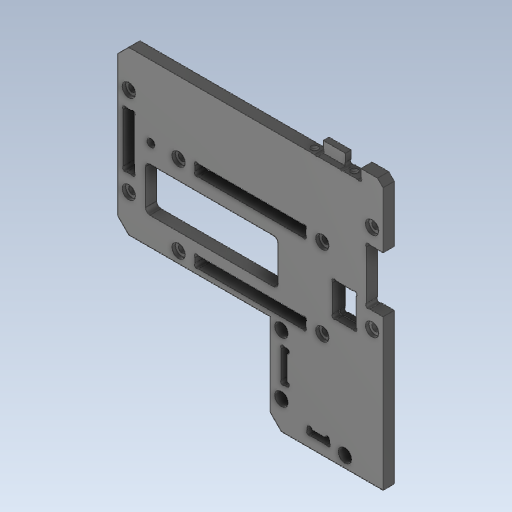
# Autodesk Inventor part: Cockpit_side_frame
Saved by Autodesk Inventor 2020.4 (Build 244396000, 396)
## iProperties
Part Number: Cockpit_side_frame
Material: アセタール樹脂、黒
Document SubType Name: Modeling
Designer: Masato Kubotera
Density: 1.425 g/cm^3
Appearance: 滑らか - 黒
Mass: 60.6497 g
Surface Area: 236.441 cm^2
Volume: 42.5612 cm^3
Description: POM T5
Author: Masato Kubotera
Autodesk Inventor part; units mm, degrees
ref_plane "YZ Plane" through (0, 0, 0) normal (1, 0, 0) x (0, 1, 0)
ref_plane "XZ Plane" through (0, 0, 0) normal (0, 1, 0) x (-1, 0, 0)
ref_plane "XY Plane" through (0, 0, 0) normal (0, 0, 1) x (1, 0, 0)
sketch "スケッチ1" plane through (0, 0, 0) normal (0, 1, 0) x (-1, 0, 0)
  line L0 (-60, 36.75) -> (60, 36.75) construction
  line L1 (60, 36.75) -> (60, -36.75) construction
  line L2 (60, -36.75) -> (-60, -36.75) construction
  line L3 (-60, -36.75) -> (-60, 36.75) construction
  line L4 (-60, 36.75) -> (60, -36.75) construction
  line L5 (60, 36.75) -> (-60, -36.75) construction
  line L6 (-52.5, 6.75) -> (52.5, 6.75) construction
  line L7 (52.5, 6.75) -> (52.5, 1.75) construction
  line L8 (52.5, 1.75) -> (-52.5, 1.75) construction
  line L9 (-52.5, 1.75) -> (-52.5, 6.75) construction
  line L10 (-52.5, 6.75) -> (52.5, 1.75) construction
  line L11 (52.5, 6.75) -> (-52.5, 1.75) construction
  line L12 (0, 36.75) -> (0, -36.75) construction
  line L13 (-57.5, 34.25) -> (-52.5, 34.25) construction
  line L14 (-52.5, 34.25) -> (-52.5, -34.25) construction
  line L15 (-52.5, -34.25) -> (-57.5, -34.25) construction
  line L16 (-57.5, -34.25) -> (-57.5, 34.25) construction
  line L17 (-57.5, 34.25) -> (-52.5, -34.25) construction
  line L18 (-52.5, 34.25) -> (-57.5, -34.25) construction
  line L19 (-55, 36.75) -> (-60, 31.75)
  line L20 (-60, 0) -> (60, 0) construction
  line L21 (-46.5, 41.75) -> (32.5, 41.75) construction
  line L22 (32.5, 41.75) -> (32.5, 11.75) construction
  line L23 (32.5, 11.75) -> (-46.5, 11.75) construction
  line L24 (-46.5, 11.75) -> (-46.5, 41.75) construction
  line L25 (-46.5, 41.75) -> (32.5, 11.75) construction
  line L26 (32.5, 41.75) -> (-46.5, 11.75) construction
  line L27 (-55, -36.75) -> (-60, -31.75)
  line L28 (-60, 31.75) -> (-60, -31.75)
  line L29 (55, -36.75) -> (60, -31.75) construction
  line L30 (-52.5, -29.25) -> (52.5, -29.25) construction
  line L31 (52.5, -29.25) -> (52.5, -34.25) construction
  line L32 (52.5, -34.25) -> (-52.5, -34.25) construction
  line L33 (-52.5, -34.25) -> (-52.5, -29.25) construction
  line L34 (-52.5, -29.25) -> (52.5, -34.25) construction
  line L35 (52.5, -29.25) -> (-52.5, -34.25) construction
  line L36 (-25, -29.25) -> (-25, -34.25) construction
  line L37 (-55, -34.25) -> (-55, 34.25) construction
  line L38 (-57.5, 12.5) -> (-52.5, 12.5) construction
  line L39 (-57.55, 12.55) -> (-52.45, 12.55)
  line L40 (-52.45, 12.55) -> (-52.45, -12.55)
  line L41 (-52.45, -12.55) -> (-57.55, -12.55)
  line L42 (-57.55, -12.55) -> (-57.55, 12.55)
  line L43 (-57.55, 12.55) -> (-52.45, -12.55) construction
  line L44 (-52.45, 12.55) -> (-57.55, -12.55) construction
  arc A0 (-52.45, 11.0651) -> (-53.9349, 12.55) centre (-53.1925, 11.8075) ccw
  circle A1 centre (-55, 20) radius 1.6
  circle A2 centre (-55, -20) radius 1.6
  arc A3 (-53.9349, -12.55) -> (-52.45, -11.0651) centre (-53.1925, -11.8075) ccw
  line L45 (-57.5, -12.5) -> (-52.5, -12.5) construction
  arc A4 (-56.0651, 12.55) -> (-57.55, 11.0651) centre (-56.8075, 11.8075) ccw
  arc A5 (-57.55, -11.0651) -> (-56.0651, -12.55) centre (-56.8075, -11.8075) ccw
  line L46 (-52.5, -31.75) -> (52.5, -31.75) construction
  line L47 (-25.05, -34.3) -> (-25.05, -29.2)
  line L48 (-25.05, -29.2) -> (25.05, -29.2)
  circle A6 centre (-32.5, -31.75) radius 1.6
  circle A7 centre (32.5, -31.75) radius 1.6
  line L49 (25, -29.25) -> (25, -34.25) construction
  line L50 (52.5, 36.75) -> (57.5, 36.75) construction
  line L51 (57.5, 36.75) -> (57.5, -34.25) construction
  line L52 (57.5, -34.25) -> (52.5, -34.25) construction
  line L53 (52.5, -34.25) -> (52.5, 36.75) construction
  line L54 (52.5, 36.75) -> (57.5, -34.25) construction
  line L55 (57.5, 36.75) -> (52.5, -34.25) construction
  line L56 (52.5, 1.25) -> (57.5, 1.25) construction
  line L57 (52.5, -11.25) -> (57.5, -11.25) construction
  line L58 (55, -34.25) -> (55, 36.75) construction
  circle A8 centre (55, -18.75) radius 1.6
  line L59 (60, -11.3) -> (52.45, -11.3)
  line L60 (52.45, -11.3) -> (52.45, 13.8)
  arc A9 (52.45, -9.8151) -> (53.9349, -11.3) centre (53.1925, -10.5575) ccw
  line L61 (52.5, 13.75) -> (57.5, 13.75) construction
  circle A10 centre (55, 21.25) radius 1.6
  line L62 (60, 13.8) -> (52.45, 13.8)
  arc A11 (53.9349, 13.8) -> (52.45, 12.3151) centre (53.1925, 13.0575) ccw
  arc A12 (-23.5651, -29.2) -> (-25.05, -30.6849) centre (-24.3075, -29.9425) ccw
  arc A13 (25.05, -30.6849) -> (23.5651, -29.2) centre (24.3075, -29.9425) ccw
  circle A14 centre (-55, 20) radius 3
  circle A15 centre (-32.5, -31.75) radius 3
  circle A16 centre (-55, -20) radius 3
  circle A17 centre (32.5, -31.75) radius 3
  line L63 (25.05, -34.3) -> (25.05, -29.2)
  line L64 (25.05, 6.8) -> (-25.05, 6.8)
  line L65 (-25.05, 6.8) -> (-25.05, 1.7)
  line L66 (-25.05, 1.7) -> (25.05, 1.7)
  line L67 (25.05, 1.7) -> (25.05, 6.8)
  line L68 (25.05, 6.8) -> (-25.05, 1.7) construction
  line L69 (-25.05, 6.8) -> (25.05, 1.7) construction
  line L70 (-25, 6.75) -> (-25, 1.75) construction
  arc A18 (-23.5651, 6.8) -> (-25.05, 5.3151) centre (-24.3075, 6.0575) ccw
  line L71 (52.5, 4.25) -> (-52.5, 4.25) construction
  circle A19 centre (-32.5, 4.25) radius 1.6
  line L72 (25, 6.75) -> (25, 1.75) construction
  arc A20 (25.05, 5.3151) -> (23.5651, 6.8) centre (24.3075, 6.0575) ccw
  circle A21 centre (32.5, 4.25) radius 1.6
  arc A22 (-25.05, 3.1849) -> (-23.5651, 1.7) centre (-24.3075, 2.4425) ccw
  arc A23 (23.5651, 1.7) -> (25.05, 3.1849) centre (24.3075, 2.4425) ccw
  line L73 (60, 31.75) -> (60, 13.8)
  line L74 (60, -11.3) -> (60, -31.75)
  circle A24 centre (-32.5, 4.25) radius 3
  circle A25 centre (55, -18.75) radius 3
  circle A26 centre (55, 21.25) radius 3
  circle A27 centre (32.5, 4.25) radius 3
  line L75 (60, 31.75) -> (60, 39.25)
  line L76 (21, 36.75) -> (-55, 36.75)
  line L77 (60, 39.25) -> (57.5, 41.75)
  line L78 (57.5, 41.75) -> (50, 41.75)
  line L79 (50, 41.75) -> (50, 36.75)
  line L80 (50, 36.75) -> (40.5, 36.75)
  line L81 (40.5, 36.75) -> (40.5, 41.75)
  line L82 (40.5, 41.75) -> (30.5, 41.75)
  line L83 (30.5, 41.75) -> (30.5, 36.75)
  line L84 (30.5, 36.75) -> (21, 36.75)
  line L85 (21, 36.75) -> (21, 36.75)
  circle A28 centre (-45, 4.25) radius 1.75
  line L86 (35.5, 41.75) -> (35.5, 36.75) construction
  line L87 (37.9, -8.6) -> (47.1, -8.6) construction
  line L88 (47.1, -8.6) -> (47.1, -22.4) construction
  line L89 (47.1, -22.4) -> (37.9, -22.4) construction
  line L90 (37.9, -22.4) -> (37.9, -8.6) construction
  line L91 (37.9, -8.6) -> (47.1, -22.4) construction
  line L92 (47.1, -8.6) -> (37.9, -22.4) construction
  line L93 (37.2, -7.95) -> (47.8, -7.95) construction
  line L94 (47.8, -7.95) -> (47.8, -23.05) construction
  line L95 (47.8, -23.05) -> (37.2, -23.05) construction
  line L96 (37.2, -23.05) -> (37.2, -7.95) construction
  line L97 (37.2, -7.95) -> (47.8, -23.05) construction
  line L98 (47.8, -7.95) -> (37.2, -23.05) construction
  line L99 (42.5, -7.95) -> (42.5, -23.05) construction
  line L100 (47.8, -15.5) -> (37.2, -15.5) construction
  line L101 (38.6349, -7.9) -> (46.3651, -7.9)
  line L102 (37.15, -9.3849) -> (37.15, -21.6151)
  line L103 (39.3349, -8.55) -> (45.6651, -8.55)
  line L104 (37.85, -10.0349) -> (37.85, -20.9651)
  arc A29 (38.6349, -7.9) -> (37.15, -9.3849) centre (37.8925, -8.6425) ccw
  arc A30 (39.3349, -8.55) -> (37.85, -10.0349) centre (38.5925, -9.2925) ccw
  arc A31 (47.85, -9.3849) -> (46.3651, -7.9) centre (47.1075, -8.6425) ccw
  arc A32 (47.15, -10.0349) -> (45.6651, -8.55) centre (46.4075, -9.2925) ccw
  line L105 (38.6349, -23.1) -> (46.3651, -23.1)
  line L106 (39.3349, -22.45) -> (45.6651, -22.45)
  arc A33 (37.15, -21.6151) -> (38.6349, -23.1) centre (37.8925, -22.3575) ccw
  arc A34 (37.85, -20.9651) -> (39.3349, -22.45) centre (38.5925, -21.7075) ccw
  arc A35 (46.3651, -23.1) -> (47.85, -21.6151) centre (47.1075, -22.3575) ccw
  arc A36 (45.6651, -22.45) -> (47.15, -20.9651) centre (46.4075, -21.7075) ccw
  line L107 (47.85, -9.3849) -> (47.85, -21.6151)
  line L108 (47.15, -10.0349) -> (47.15, -20.9651)
  line L109 (-45.5, -4.25) -> (10.5, -4.25)
  line L110 (12.5, -6.25) -> (12.5, -22.25)
  line L111 (10.5, -24.25) -> (-45.5, -24.25)
  line L112 (-47.5, -22.25) -> (-47.5, -6.25)
  line L113 (-47.5, -4.25) -> (12.5, -24.25) construction
  line L114 (12.5, -4.25) -> (-47.5, -24.25) construction
  arc A37 (-45.5, -4.25) -> (-47.5, -6.25) centre (-45.5, -6.25) ccw
  arc A38 (-47.5, -22.25) -> (-45.5, -24.25) centre (-45.5, -22.25) ccw
  arc A39 (10.5, -24.25) -> (12.5, -22.25) centre (10.5, -22.25) ccw
  arc A40 (12.5, -6.25) -> (10.5, -4.25) centre (10.5, -6.25) ccw
  line L115 (26.5, 36.75) -> (26.5, 32.75) construction
  line L116 (24.5, 32.75) -> (28.5, 32.75) construction
  line L117 (28.5, 32.75) -> (28.5, 36.75) construction
  line L118 (24.5, 32.75) -> (24.5, 36.75) construction
  line L119 (44.5, 36.75) -> (44.5, 32.75) construction
  line L120 (46.5, 32.75) -> (42.5, 32.75) construction
  line L121 (42.5, 32.75) -> (42.5, 36.75) construction
  line L122 (46.5, 32.75) -> (46.5, 36.75) construction
  arc A41 (48.5151, 36.75) -> (50, 38.2349) centre (49.2575, 37.4925) ccw
  arc A42 (29.0151, 36.75) -> (30.5, 38.2349) centre (29.7575, 37.4925) ccw
  arc A43 (40.5, 38.2349) -> (41.9849, 36.75) centre (41.2425, 37.4925) ccw
  line L123 (30.5, 36.75) -> (40.5, 36.75)
  line L124 (60, -36.75) -> (60, -79.25)
  line L125 (60, -79.25) -> (14, -79.25)
  line L126 (9, -74.25) -> (9, -36.75)
  arc A44 (-25.05, -32.8151) -> (-23.5651, -34.3) centre (-24.3075, -33.5575) ccw
  arc A45 (23.5651, -34.3) -> (25.05, -32.8151) centre (24.3075, -33.5575) ccw
  line L127 (60, -36.75) -> (60, -31.75)
  line L128 (-25.05, -34.3) -> (25.05, -34.3)
  line L129 (-55, -36.75) -> (9, -36.75)
  line L130 (16.5, -48.75) -> (50.5, -48.75) construction
  line L131 (50.5, -48.75) -> (50.5, -71.75) construction
  line L132 (50.5, -71.75) -> (16.5, -71.75) construction
  line L133 (16.5, -71.75) -> (16.5, -48.75) construction
  line L134 (16.5, -48.75) -> (50.5, -71.75) construction
  line L135 (50.5, -48.75) -> (16.5, -71.75) construction
  line L136 (14, -45.5) -> (16.5, -45.5) construction
  line L137 (16.5, -45.5) -> (16.5, -60.5) construction
  line L138 (16.5, -60.5) -> (14, -60.5) construction
  line L139 (14, -60.5) -> (14, -45.5) construction
  line L140 (14, -45.5) -> (16.5, -60.5) construction
  line L141 (16.5, -45.5) -> (14, -60.5) construction
  line L142 (13.95, -45.45) -> (16.55, -45.45)
  line L143 (16.55, -45.45) -> (16.55, -60.55)
  line L144 (16.55, -60.55) -> (13.95, -60.55)
  line L145 (13.95, -60.55) -> (13.95, -45.45)
  line L146 (13.95, -45.45) -> (16.55, -60.55) construction
  line L147 (16.55, -45.45) -> (13.95, -60.55) construction
  line L148 (15.25, -45.5) -> (15.25, -60.5) construction
  line L149 (14, -53) -> (16.5, -53) construction
  arc A46 (15.4349, -45.45) -> (13.95, -46.9349) centre (14.6925, -46.1925) ccw
  arc A47 (16.55, -47.55) -> (16.55, -45.45) centre (16.55, -46.5) ccw
  arc A48 (13.95, -59.0651) -> (15.4349, -60.55) centre (14.6925, -59.8075) ccw
  arc A49 (16.55, -60.55) -> (16.55, -58.45) centre (16.55, -59.5) ccw
  line L150 (11.5, -34.25) -> (16.5, -34.25) construction
  line L151 (16.5, -34.25) -> (16.5, -71.75) construction
  line L152 (16.5, -71.75) -> (11.5, -71.75) construction
  line L153 (11.5, -71.75) -> (11.5, -34.25) construction
  line L154 (11.5, -34.25) -> (16.5, -71.75) construction
  line L155 (16.5, -34.25) -> (11.5, -71.75) construction
  circle A50 centre (14, -39.5) radius 1.6
  line L156 (14, -34.25) -> (14, -71.75) construction
  circle A51 centre (14, -66.5) radius 1.6
  line L157 (14, -79.25) -> (9, -74.25)
  circle A52 centre (14, -39.5) radius 3
  circle A53 centre (14, -66.5) radius 3
  line L158 (11.5, -71.75) -> (50, -71.75) construction
  line L159 (50, -71.75) -> (50, -76.75) construction
  line L160 (50, -76.75) -> (11.5, -76.75) construction
  line L161 (11.5, -76.75) -> (11.5, -71.75) construction
  line L162 (11.5, -71.75) -> (50, -76.75) construction
  line L163 (50, -71.75) -> (11.5, -76.75) construction
  line L164 (30.75, -76.75) -> (30.75, -71.75) construction
  line L165 (11.5, -74.25) -> (50, -74.25) construction
  line L166 (25.75, -71.75) -> (35.75, -71.75) construction
  line L167 (35.75, -71.75) -> (35.75, -74.25) construction
  line L168 (35.75, -74.25) -> (25.75, -74.25) construction
  line L169 (25.75, -74.25) -> (25.75, -71.75) construction
  line L170 (25.75, -71.75) -> (35.75, -74.25) construction
  line L171 (35.75, -71.75) -> (25.75, -74.25) construction
  line L172 (25.7, -71.7) -> (35.8, -71.7)
  line L173 (35.8, -71.7) -> (35.8, -74.3)
  line L174 (35.8, -74.3) -> (25.7, -74.3)
  line L175 (25.7, -74.3) -> (25.7, -71.7)
  line L176 (25.7, -71.7) -> (35.8, -74.3) construction
  line L177 (35.8, -71.7) -> (25.7, -74.3) construction
  arc A54 (25.7, -72.8151) -> (27.1849, -74.3) centre (26.4425, -73.5575) ccw
  arc A55 (27.8, -71.7) -> (25.7, -71.7) centre (26.75, -71.7) ccw
  arc A56 (34.3151, -74.3) -> (35.8, -72.8151) centre (35.0575, -73.5575) ccw
  arc A57 (35.8, -71.7) -> (33.7, -71.7) centre (34.75, -71.7) ccw
  circle A58 centre (42.75, -74.25) radius 1.6
  circle A59 centre (42.75, -74.25) radius 3
  point P0 (0, 0)
  point P1 (0, 4.25)
  point P2 (-55, 0)
  point P3 (-55, 0)
  point P4 (-7, 26.75)
  point P5 (0, -31.75)
  point P6 (-25.05, -34.25)
  point P7 (25.05, -34.25)
  point P8 (0, 4.25)
  point P9 (52.45, 12.3151)
  point P10 (25.05, 3.1849)
  point P11 (23.5651, 1.7)
  point P12 (-23.5651, 1.7)
  point P13 (-25.05, 3.1849)
  point P14 (23.5651, 6.8)
  point P15 (25.05, 5.3151)
  point P16 (-57.55, -11.0651)
  point P17 (-57.55, 11.0651)
  point P18 (-56.0651, 12.55)
  point P19 (-52.45, -11.0651)
  point P20 (-53.9349, -12.55)
  point P21 (-56.0651, -12.55)
  point P22 (42.5, -15.5)
  point P23 (37.15, -7.9)
  point P24 (37.85, -8.55)
  point P25 (-17.5, -14.25)
  point P26 (41.9849, 36.75)
  point P27 (9, -79.25)
  point P28 (-23.5651, -34.3)
  point P29 (25.05, -32.8151)
  point P30 (33.5, -60.25)
  point P31 (15.25, -53)
  point P32 (30.75, -74.25)
  point P33 (30.75, -73)
  point P34 (33.7, -71.7)
  point P35 (35.8, -72.8151)
  point P36 (16.55, -58.45)
  point P37 (15.4349, -60.55)
  dimension "d0" = 73.5
  dimension "d1" = 120
  dimension "d3" = 5
  dimension "d4" = 5
  dimension "d6" = 5
  dimension "d7" = 5
  dimension "d8" = 79
  dimension "d9" = 6
  dimension "d11" = 5
  dimension "d12" = 1.05
  dimension "d13" = 3.2
  dimension "d14" = 40
  dimension "d15" = 25
  dimension "d16" = 0.05
  dimension "d17" = 0.05
  dimension "d18" = 3.2
  dimension "d19" = 50
  dimension "d20" = 0.05
  dimension "d21" = 0.05
  dimension "d23" = 65
  dimension "d24" = 5
  dimension "d25" = 30
  dimension "d28" = 3.2
  dimension "d29" = 1.05
  dimension "d30" = 0.05
  dimension "d31" = 0.05
  dimension "d32" = 40
  dimension "d33" = 25
  dimension "d34" = 105
  dimension "d35" = 1.05
  dimension "d36" = 5
  dimension "d37" = 5
  dimension "d38" = 6
  dimension "d39" = 6
  dimension "d41" = 1.05
  dimension "d42" = 3.2
  dimension "d43" = 50
  dimension "d44" = 0.05
  dimension "d45" = 0.05
  dimension "d46" = 65
  dimension "d47" = 31
  dimension "d51" = 6
  dimension "d52" = 6
  dimension "d55" = 68.5
  dimension "d63" = 20
  dimension "d64" = 5
  dimension "d66" = 3.5
  dimension "d69" = 32.5
  dimension "d70" = 10
  dimension "d72" = 2.5
  dimension "d73" = 2.5
  dimension "d74" = 10
  dimension "d75" = 14.5
  dimension "d76" = 81
  dimension "d77" = 9.2
  dimension "d78" = 13.8
  dimension "d79" = 10.6
  dimension "d80" = 15.1
  dimension "d84" = 1.05
  dimension "d85" = 0.05
  dimension "d86" = 0.05
  dimension "d87" = 0.05
  dimension "d88" = 0.05
  dimension "d89" = 1.05
  constraints: 356 end point, 94 symmetric about line, 87 point on circle, 72 point on line, 69 midpoint, 60 centre point, 44 parallel, 33 perpendicular, 19 horizontal, 13 collinear, 8 tangent, 6 coincident, 4 vertical, 3 equal radius, 31 other
  measures "d0" distance of L0.end L1.end
  measures "d1" distance of L0.start L0.end
  measures "d3" distance of L6.end L7.end
  measures "d4" distance of L13.start L13.end
  measures "d6" distance of L0.start L19.start
  measures "d7" distance of L19.end L0.start
  measures "d8" distance of L21.start L21.end
  measures "d9" distance between parallel lines of L14 L24
  measures "d11" distance of L30.end L31.end
  measures "d12" radius of A0
  measures "d13" diameter of A1
  measures "d14" distance of A2.centre A1.centre
  measures "d15" distance between parallel lines of L45 L38
  measures "d16" distance between parallel lines of L38 L39
  measures "d17" distance between parallel lines of L42 L16
  measures "d18" diameter of A6
  measures "d19" distance of L49.end L36.end
  measures "d20" distance between parallel lines of L47 L36
  measures "d21" distance between parallel lines of L30 L48
  measures "d23" distance of A7.centre A6.centre
  measures "d24" distance of L51.end L52.end
  measures "d25" distance of L21.end L22.end
  measures "d28" diameter of A8
  measures "d29" radius of A9
  measures "d30" distance between parallel lines of L60 L53
  measures "d31" distance between parallel lines of L61 L62
  measures "d32" distance of A8.centre A10.centre
  measures "d33" distance between parallel lines of L57 L61
  measures "d34" distance of L7.end L8.end
  measures "d35" radius of A12
  measures "d36" distance between parallel lines of L21 L0
  measures "d37" distance between parallel lines of L6 L23
  measures "d38" diameter of A14
  measures "d39" diameter of A15
  measures "d41" radius of A18
  measures "d42" diameter of A19
  measures "d43" distance between parallel lines of L72 L70
  measures "d44" distance between parallel lines of L65 L70
  measures "d45" distance between parallel lines of L64 L6
  measures "d46" distance of A21.centre A19.centre
  measures "d47" distance of L30.start L8.end
  measures "d51" diameter of A24
  measures "d52" diameter of A25
  measures "d55" distance of L15.end L13.start
  measures "d63" distance between parallel lines of L22 L53
  measures "d64" distance of L83.end L82.end
  measures "d66" diameter of A28
  measures "d69" vertical distance of A28.centre L0.start
  measures "d70" distance of L81.end L82.end
  measures "d72" horizontal distance of L75.end L77.end
  measures "d73" horizontal distance of L75.end L77.end
  measures "d74" horizontal distance of L78.end L75.end
  measures "d75" horizontal distance of L84.end L86.start
  measures "d76" distance of L0.start L84.end
  measures "d77" distance of L88.end L89.end
  measures "d78" distance of L87.end L88.end
  measures "d79" distance of L94.end L95.end
  measures "d80" distance of L93.end L94.end
  measures "d84" radius of A29
  measures "d85" distance between parallel lines of L93 L101
  measures "d86" distance between parallel lines of L102 L96
  measures "d87" distance between parallel lines of L87 L103
  measures "d88" distance between parallel lines of L104 L90
  measures "d89" radius of A30
extrude "押し出し1" add sketch "スケッチ1" along normal blind 5 contours L76 L84 A42 L123 A43 L80 A41 L79 L78 L77 L75 L73 L62 A11 L60 A9 L59 L74 L127 L124 L125 L157 L126 L129 L27 L28 L19
extrude "押し出し2" add sketch "スケッチ1" along normal blind 3.5 contours A14 | A15 | A16 | A17 | A24 | A25 | A26 | A27
extrude "押し出し3" add sketch "スケッチ1" along normal blind 2 contours L101 A31 L107 A35 L105 A33 L102 A29
extrude "押し出し4" add sketch "スケッチ1" along normal blind 2.5 contours A42 L83 L82 L81 A43 L123
sketch "スケッチ2" plane through (-30.5, 0, 36.75) normal (0, 0, 1) x (1, 0, 0)
  line L0 (-14, 2.5) -> (4, 2.5)
  line L1 (-10, 0) -> (0, 0) projected
  line L2 (-5, 0) -> (-5, 5)
  line L3 (-10, 5) -> (0, 5) projected
  point P0 (30.5, 0)
  point P1 (-5, 2.5)
  dimension "d104" = 18
  constraints: 4 end point, 4 midpoint, 1 horizontal, 1 symmetric about line
  measures "d104" distance of L0.end L0.start
hole "穴1" at (-26.5, 2.5, 36.75) at (-44.5, 2.5, 36.75) direction (0, 0, -1) diameter 3.242 depth 11.8 tip angle 118 thread size "M4x0.7" class "6H" standard "ISO Metric profile"
equation "\"d7\" = d6"
equation "\"d18\" = d13"
equation "\"d20\" = d16"
equation "\"d21\" = d20"
equation "\"d29\" = d12"
equation "\"d30\" = d16"
equation "\"d31\" = d30"
equation "\"d35\" = d12"
